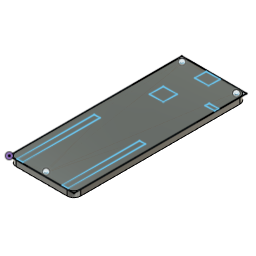
jtagulator case v6 (Autodesk Fusion 360 design; units mm, degrees)
Autodesk Fusion 360 part; units mm, degrees
sketch "Sketch1" plane through (0, 0, 0) normal (0, 0, 1) x (1, 0, 0)
  line L0 (0, 0) -> (57.1, 0)
  line L1 (57.1, 0) -> (57.1, 152.3)
  line L2 (57.1, 152.3) -> (0, 152.3)
  line L3 (0, 152.3) -> (0, 0)
  circle A0 centre (28.5, 4) radius 1.2512
  circle A1 centre (52.5, 148) radius 1.2512
  circle A2 centre (4.5, 148) radius 1.2512
  line L4 (6, 69) -> (11, 69)
  line L5 (11, 69) -> (11, 1)
  line L6 (11, 1) -> (6, 1)
  line L7 (6, 1) -> (6, 69)
  line L8 (46, 1) -> (46, 69)
  line L9 (46, 69) -> (51, 69)
  line L10 (51, 69) -> (51, 1)
  line L11 (51, 1) -> (46, 1)
  line L12 (15, 121) -> (27, 121)
  line L13 (27, 121) -> (27, 109)
  line L14 (27, 109) -> (15, 109)
  line L15 (15, 109) -> (15, 121)
  line L16 (48.19, 128.3216) -> (56.4181, 128.3216)
  line L17 (56.4181, 128.3216) -> (56.4181, 124.9122)
  line L18 (56.4181, 124.9122) -> (48.19, 124.9122)
  line L19 (48.19, 124.9122) -> (48.19, 128.3216)
  line L20 (22.55, 151.4) -> (34.55, 151.4)
  line L21 (34.55, 151.4) -> (34.55, 141.4)
  line L22 (34.55, 141.4) -> (22.55, 141.4)
  line L23 (22.55, 141.4) -> (22.55, 151.4)
  dimension "d1" = 57.1
  dimension "d2" = 152.3
  dimension "d6" = 5
  dimension "d7" = 68
  dimension "d8" = 5
  dimension "d9" = 68
  dimension "d10" = 12
  dimension "d13" = 12
  dimension "d14" = 10
  constraint horizontal L0
  constraint vertical L1
  constraint horizontal L2
  constraint vertical L3
  constraint coincident L0.start L3.end
  constraint horizontal L4
  constraint vertical L5
  constraint horizontal L6
  constraint vertical L7
  constraint horizontal L9
  constraint vertical L10
  constraint horizontal L11
  constraint vertical L8
  constraint horizontal L12
  constraint vertical L13
  constraint horizontal L14
  constraint vertical L15
  constraint horizontal L16
  constraint vertical L17
  constraint horizontal L18
  constraint vertical L19
  constraint horizontal L20
  constraint vertical L21
  constraint horizontal L22
  constraint vertical L23
  measures "d1" distance of L0.start L0.end
  measures "d2" distance of L0.start L2.end
  measures "d6" distance of L4.start L4.end
  measures "d7" distance of L4.start L6.end
  measures "d8" distance of L9.end L8.end
  measures "d9" distance of L8.end L8.start
  measures "d10" distance of L12.start L12.end
  measures "d13" distance of L20.start L20.end
  measures "d14" distance of L20.start L22.end
extrude "Extrude1" add sketch "Sketch1" against normal blind 2.5 contours L8 L9 L10 L11 makes body 1
extrude "Extrude2" add sketch "Sketch1" against normal blind 2.5 separate body contours L4 L5 L6 L7 makes body 2
extrude "Extrude3" add sketch "Sketch1" against normal blind 2.5 separate body contours L12 L13 L14 L15 makes body 3
extrude "Extrude4" add sketch "Sketch1" against normal blind 2.5 separate body contours L16 L17 L18 L19 makes body 4
extrude "Extrude5" add sketch "Sketch1" against normal blind 2.5 separate body contours L20 L21 L22 L23 makes body 5
extrude "Extrude6" add sketch "Sketch1" against normal blind 4 bodies 1 2 3 4 5
extrude "Extrude7" add 1 faces at (28.5262, 47.7496, -4) along direction (0, 0, -1) blind 1.2 on bodies 1 bodies 1
extrude "Extrude8" add 1 faces at (19.0333, 152.3, -3.4667) along direction (0, 1, 0) blind 0.25 on bodies 1 bodies 1
fillet "Fillet5" radius 6 4 edges at (57.1, 0, -2.6) (0, 0, -2.6) (0, 152.55, -2.6) (57.1, 152.55, -2.6) on bodies 1
